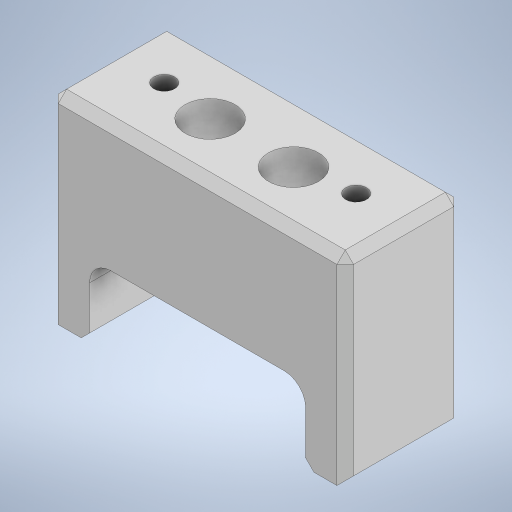
# Autodesk Inventor part: BK12_Spacer
Saved by Autodesk Inventor 2023 (Build 270158000, 158)
## iProperties
Created: 2022-05-04
Part Number: BK12_Spacer
Material: Generic
Document SubType Name: Modeling
Designer: plebbb
Density: 1 g/cm^3
Appearance: Default
Mass: 113.997 g
Surface Area: 238.823 cm^2
Volume: 113.997 cm^3
Author: plebbb
Autodesk Inventor part; units mm, degrees
note: some values were not read from the file. Chosen so that the rebuilt part matches the saved one: second side of "Extrusion1".
ref_plane "YZ Plane" through (0, 0, 0) normal (1, 0, 0) x (0, 1, 0)
ref_plane "XZ Plane" through (0, 0, 0) normal (0, 1, 0) x (-1, 0, 0)
sketch "Sketch1" plane through (0, 0, 0) normal (0, 1, 0) x (-1, 0, 0)
  line L0 (0, 0) -> (60, 0) construction
  line L1 (60, 0) -> (60, -20) construction
  line L2 (60, -20) -> (0, -20) construction
  line L3 (0, -20) -> (0, 0) construction
  line L4 (60.5, 0.5) -> (-0.5, 0.5)
  line L5 (-0.5, 0.5) -> (-0.5, -20.5)
  line L6 (-0.5, -20.5) -> (60.5, -20.5)
  line L7 (60.5, -20.5) -> (60.5, 0.5)
  circle A0 centre (53, -12) radius 2.5
  circle A1 centre (7, -12) radius 2.5
  line L8 (53, -12) -> (7, -12) construction
  point P0 (30, -12)
  point P1 (30, -20)
  point P2 (0, -10)
  point P3 (-0.5, -10)
  dimension "d0" = 20
  dimension "d1" = 60
  dimension "d2" = 0.5
  dimension "d3" = 0.5
  dimension "d4" = 0.5
  dimension "d5" = 0.5
  dimension "d6" = 5
  dimension "d7" = 46
  dimension "d109" = 2
  constraints: 18 end point, 4 midpoint, 4 parallel, 3 horizontal, 2 centre point, 2 coincident, 2 perpendicular, 1 equal radius, 1 vertical alignment
  measures "d0" distance of L0.end L1.end
  measures "d1" distance of L1.end L2.end
  measures "d2" distance between parallel lines of L7 L1
  measures "d3" distance between parallel lines of L5 L3
  measures "d4" distance between parallel lines of L6 L2
  measures "d5" distance between parallel lines of L4 L0
  measures "d6" diameter of A0
  measures "d7" distance of L8.start L8.end
  measures "d109" vertical distance of point (-0.5, -10) L8.end
sketch "Sketch2" plane through (0, 0, 0) normal (0, 1, 0) x (-1, 0, 0)
  line L0 (-5.4, 5) -> (65.4, 5)
  line L1 (65.4, 5) -> (65.4, -25)
  line L2 (65.4, -25) -> (-5.4, -25)
  line L3 (-5.4, -25) -> (-5.4, 5)
  line L4 (60.5, -20.5) -> (60.5, 0.5) construction
  line L5 (-0.5, 0.5) -> (-0.5, -20.5) construction
  line L6 (-0.5, -20.5) -> (60.5, -20.5) construction
  point P0 (0, 0)
  point P1 (60.5, -10)
  point P2 (65.4, -10)
  point P3 (30, -20.5)
  point P4 (30, -25)
  dimension "d9" = 70.8
  dimension "d10" = 30
  dimension "d44" = 35.4
  constraints: 8 end point, 4 midpoint, 2 parallel, 1 horizontal, 1 horizontal alignment, 1 perpendicular
  measures "d9" distance of L1.end L2.end
  measures "d10" distance of L0.end L1.end
  measures "d44" distance from line of L1 point (30, -20.5)
extrude "Extrusion1" add sketch "Sketch2" against normal blind 30.4
extrude "Extrusion3" cut sketch "Sketch1" against normal blind 43.3375 and the other way blind 30.4 contours A0 | A1
sketch "Sketch3" plane through (5.4, -30.4, -25) normal (0, 0, -1) x (1, 0, 0)
  line L0 (-70.8, 0) -> (0, 0) projected
  line L1 (0, 0) -> (0, 17.5)
  line L2 (0, 17.5) -> (-9.5, 17.5)
  line L3 (-9.5, 17.5) -> (-9.5, 5.08)
  line L4 (-14.58, 0) -> (-56.22, 0)
  line L5 (-61.3, 5.08) -> (-61.3, 17.5)
  line L6 (-61.3, 17.5) -> (-70.8, 17.5)
  line L7 (-70.8, 17.5) -> (-70.8, 0)
  arc A0 (-14.58, 0) -> (-9.5, 5.08) centre (-14.58, 5.08) ccw
  arc A1 (-61.3, 5.08) -> (-56.22, 0) centre (-56.22, 5.08) ccw
  point P0 (-9.5, 0)
  point P1 (-61.3, 0)
  point P2 (-61.3, 11.29)
  point P3 (-9.5, 11.29)
  point P4 (-4.75, 17.5)
  dimension "d94" = 51.8
  dimension "d95" = 17.5
  dimension "d96" = 5.08
  constraints: 14 end point, 6 point on line, 4 perpendicular, 4 point on circle, 4 tangent, 3 midpoint, 2 centre point, 2 equal length, 2 vertical, 1 equal radius
  measures "d94" distance of point (-61.3, 11.29) point (-9.5, 11.29)
  measures "d95" distance from line of L0 point (-4.75, 17.5)
  measures "d96" radius of A0
extrude "Extrusion4" add sketch "Sketch3" against normal up to surface (30 mm away)
ref_plane "Work Plane3" through (-49.05, -33.575, -1214.2) normal (0, -1, 0) x (1, 0, 0)
sketch "Sketch4" plane through (0, 0, 0) normal (0, 1, 0) x (1, 0, 0)
  line L0 (-60.5, 20.5) -> (0.5, 20.5) construction
  line L1 (-60.5, -0.5) -> (-60.5, 20.5) construction
  circle A0 centre (-40, 10) radius 3
  line L2 (5.4, 25) -> (-65.4, 25) projected
  line L3 (-65.4, 25) -> (-65.4, -5) projected
  circle A1 centre (-20, 10) radius 3
  line L4 (-40, 10) -> (-20, 10) construction
  point P0 (0, 0)
  point P1 (-30, 20.5)
  point P2 (-60.5, 10)
  point P3 (-65.4, 20.5)
  point P4 (5.4, 20.5)
  point P5 (-30, 20.5)
  point P6 (-60.5, 10)
  point P7 (-65.4, 10)
  point P8 (-30, 25)
  point P9 (-30, 10)
  dimension "d82" = 6
  dimension "d98" = 20
  dimension "d107" = 0
  constraints: 7 midpoint, 6 end point, 2 centre point, 2 horizontal, 2 vertical alignment, 1 equal radius, 1 horizontal alignment, 1 vertical, 2 other
  measures "d82" diameter of A0
  measures "d98" distance of L4.start L4.end
  measures "d107" vertical distance of point (-60.5, 10) point (-30, 10)
extrude "Extrusion5" cut sketch "Sketch4" against normal up to surface (33.575 mm away)
extrude "Extrusion2" cut sketch "Sketch1" against normal blind 43.3375 and the other way blind 5 contours A0 | A1
sketch "Sketch8" plane through (15.4, 40, -25) normal (0, 0, -1) x (1, 0, 0)
  line L0 (25.4, 30) -> (34.4, 30)
  line L1 (34.4, 30) -> (35.4, 31)
  line L2 (35.4, 31) -> (35.4, 34)
  line L3 (35.4, 34) -> (31.95, 37.45)
  line L4 (31.95, 37.45) -> (31.95, 39.8767)
  line L5 (31.95, 39.8767) -> (33.1672, 41.0939)
  arc A0 (34.8792, 42.8058) -> (33.1672, 41.0939) centre (35.1489, 40.8241) ccw
  line L6 (34.8792, 42.8058) -> (35.4, 43.3267)
  line L7 (35.4, 43.3267) -> (35.4, 44.66)
  line L8 (35.4, 44.66) -> (34.8792, 45.1808)
  arc A1 (33.1672, 46.8928) -> (34.8792, 45.1808) centre (35.1489, 47.1626) ccw
  line L9 (33.1672, 46.8928) -> (32.56, 47.5)
  line L10 (32.56, 47.5) -> (25.4, 47.5)
  line L11 (25.4, 47.5) -> (25.4, 30) construction
  line L12 (33.1672, 41.0939) -> (34.8792, 42.8058) construction
  line L13 (33.1672, 46.8928) -> (34.8792, 45.1808) construction
  line L14 (25.4, 30) -> (16.4, 30)
  line L15 (16.4, 30) -> (15.4, 31)
  line L16 (15.4, 31) -> (15.4, 34)
  line L17 (15.4, 34) -> (18.85, 37.45)
  line L18 (18.85, 37.45) -> (18.85, 39.8767)
  line L19 (18.85, 39.8767) -> (17.6328, 41.0939)
  arc A2 (17.6328, 41.0939) -> (15.9208, 42.8058) centre (15.6511, 40.8241) ccw
  line L20 (15.9208, 42.8058) -> (15.4, 43.3267)
  line L21 (15.4, 43.3267) -> (15.4, 44.66)
  line L22 (15.4, 44.66) -> (15.9208, 45.1808)
  arc A3 (15.9208, 45.1808) -> (17.6328, 46.8928) centre (15.6511, 47.1626) ccw
  line L23 (17.6328, 46.8928) -> (18.24, 47.5)
  line L24 (18.24, 47.5) -> (25.4, 47.5)
  line L25 (17.6328, 41.0939) -> (15.9208, 42.8058) construction
  line L26 (17.6328, 46.8928) -> (15.9208, 45.1808) construction
  arc A4 (50.8, 26.825) -> (47.625, 30) centre (47.625, 26.825) ccw construction
  line L27 (34.4, 30) -> (35.4, 30)
  line L28 (3.175, 30) -> (47.625, 30) projected
  line L29 (35.4, 31) -> (35.4, 30)
  line L30 (15.4, 31) -> (15.4, 30)
  line L31 (15.4, 30) -> (16.4, 30)
  point P0 (-15.4, 40)
  point P1 (35.4, 32.5)
  dimension "d64" = 1
  dimension "d65" = 3
  dimension "d66" = 135
  dimension "d67" = 2
  dimension "d69" = 3.45
  dimension "d71" = 17.5
  dimension "d72" = 7.16
  dimension "d73" = 2.375
  dimension "d74" = 1.3333
  dimension "d75" = 2.4211
  dimension "d76" = 15.4
  dimension "d77" = 10
  constraints: 62 end point, 14 symmetric about line, 8 point on circle, 6 perpendicular, 4 centre point, 4 collinear, 3 vertical alignment, 2 horizontal, 2 parallel, 2 vertical, 1 equal radius, 1 horizontal alignment, 1 midpoint, 1 point on line, 2 other
  measures "d64" distance from line of L0 L1.end
  measures "d65" distance of L1.end L2.end
  measures "d66" angle of L2 L3
  measures "d67" radius of A1
  measures "d69" horizontal distance of L3.end L2.end
  measures "d71" distance of L10.end L0.start
  measures "d72" distance of L9.end L10.end
  measures "d73" distance of L6.start L8.end
  measures "d74" distance of L6.end L7.end
  measures "d75" distance of L5.end L6.start
  measures "d76" horizontal distance of A4.start point (35.4, 32.5)
  measures "d77" horizontal distance of L0.start L1.end
extrude "Extrusion8" [suppressed]
thicken "Thicken1" [suppressed]
sketch "Sketch11" plane through (0, 0, 0) normal (0, 1, 0) x (1, 0, 0)
  circle A0 centre (-20, 10) radius 6
  circle A1 centre (-40, 10) radius 3 projected
  circle A2 centre (-20, 10) radius 3 projected
  circle A3 centre (-40, 10) radius 6
  point P0 (0, 0)
  dimension "d99" = 12
  constraints: 2 centre point, 2 concentric, 1 equal radius
  measures "d99" diameter of A3
extrude "Extrusion11" cut sketch "Sketch11" against normal blind 10 contours A0 | A1 | A2 | A3
sketch "Sketch12" plane through (-50.82, -30.4, 5) normal (0, 0, 1) x (1, 0, 0)
  line L0 (-31.8767, 47.5596) -> (80.4706, 47.5596)
  line L1 (80.4706, 47.5596) -> (80.4706, -43.9783)
  line L2 (80.4706, -43.9783) -> (-31.8767, -43.9783)
  line L3 (-31.8767, -43.9783) -> (-31.8767, 47.5596)
  point P0 (50.82, 30.4)
  constraints: 8 end point, 2 parallel, 1 horizontal, 1 perpendicular
extrude "Extrusion12" cut sketch "Sketch12" against normal blind 2
chamfer "Chamfer1" distance 2 angle 45 12 edges at (5.4, 0, -11) (-30, 0, -25) (5.4, -23.95, -25) (-65.4, -23.95, -25) (-55.9, -47.9, -11) (5.4, -47.9, -11) (-65.4, 0, -11) (-65.4, -47.9, -11) (-4.1, -47.9, -11) (-30, 0, 3) (-65.4, -23.95, 3) (5.4, -23.95, 3)
body "Solid1"
